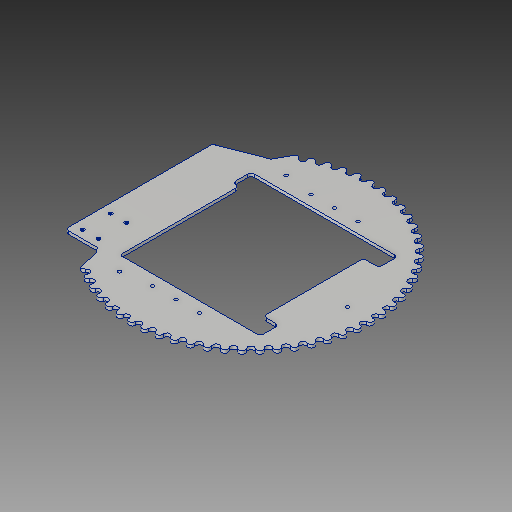
# Autodesk Inventor part: Bearing Plate
Saved by Autodesk Inventor 2019.4 (Build 234330000, 330)
## iProperties
Created: 2020-01-22
Part Number: Bearing Plate
Material: Aluminum 6061
Document SubType Name: Modeling
Designer: admin
Density: 2.7 g/cm^3
Appearance: Aluminum - Flat
Mass: 922.466 g
Surface Area: 1512.08 cm^2
Volume: 341.654 cm^3
Author: admin
Autodesk Inventor part; units mm, degrees
ref_plane "YZ Plane" through (0, 0, 0) normal (1, 0, 0) x (0, 1, 0)
ref_plane "XZ Plane" through (0, 0, 0) normal (0, 1, 0) x (-1, 0, 0)
ref_plane "XY Plane" through (0, 0, 0) normal (0, 0, 1) x (1, 0, 0)
sketch "Sketch1" plane through (0, 0, 0) normal (0, 1, 0) x (-1, 0, 0)
  arc A0 (63.1453, -163.2105) -> (129.2323, 118) centre (0, 0) ccw construction
  circle A1 centre (0, 0) radius 101.6 construction
  line L0 (-100.2, 110.3) -> (100.2, 110.3)
  line L1 (100.2, 110.3) -> (100.2, -110.3)
  line L2 (100.2, -110.3) -> (-100.2, -110.3)
  line L3 (-100.2, -110.3) -> (-100.2, 110.3)
  line L4 (-100.2, 110.3) -> (100.2, -110.3) construction
  line L5 (100.2, 110.3) -> (-100.2, -110.3) construction
  line L6 (180, 118) -> (180, -118)
  line L7 (180, -118) -> (63.1453, -163.2105)
  line L8 (180, 0) -> (0, 0)
  line L9 (180, 118) -> (129.2323, 118)
  arc A2 (129.2323, 118) -> (63.1453, -163.2105) centre (0, 0) ccw
  dimension "d0" = 350
  dimension "d1" = 203.2
  dimension "d4" = 220.6
  dimension "d5" = 200.4
  dimension "d6" = 180
  dimension "d7" = 118
  constraints: 20 end point, 4 point on circle, 3 centre point, 3 midpoint, 2 coincident, 2 horizontal, 2 parallel, 2 perpendicular, 1 tangent, 1 vertical
  measures "d0" diameter of A0
  measures "d1" diameter of A1
  measures "d4" distance of L2.end L0.start
  measures "d5" distance of L0.start L0.end
  measures "d6" distance from line of point (0, 0) L6
  measures "d7" distance from line of point (0, 0) L9
extrude "Extrusion1" add sketch "Sketch1" along normal blind 5
sketch "Sketch2" plane through (0, 0, 0) normal (0, -1, 0) x (1, 0, 0)
  circle A0 centre (-165.208, 60.275) radius 2.0193 construction
  circle A1 centre (-165.208, 105.1064) radius 2.0193 construction
  circle A2 centre (-139.808, 105.1064) radius 2.0193 construction
  circle A3 centre (-139.808, 60.275) radius 2.0193 construction
  circle A4 centre (-165.208, 105.1064) radius 3
  circle A5 centre (-139.808, 105.1064) radius 3
  circle A6 centre (-139.808, 60.275) radius 3
  circle A7 centre (-165.208, 60.275) radius 3
  point P0 (0, 0)
  dimension "d75" = 6
  dimension "d76" = 6
  dimension "d77" = 6
  dimension "d78" = 6
  constraints: 4 centre point, 4 coincident
  measures "d75" diameter of A4
  measures "d76" diameter of A5
  measures "d77" diameter of A6
  measures "d78" diameter of A7
extrude "Extrusion2" cut sketch "Sketch2" against normal through all
chamfer "Chamfer1" distance 3 angle 45 4 edges at (-168.208, 0, 60.275) (-142.808, 0, 60.275) (-142.808, 0, 105.1064) (-168.208, 0, 105.1064)
sketch "Sketch3" plane through (0, 5, 0) normal (0, 1, 0) x (1, 0, 0)
  line L0 (154.73, 0) -> (-77.365, -134.0001) construction
  line L1 (-77.365, -134.0001) -> (-77.365, 134.0001) construction
  line L2 (-77.365, 134.0001) -> (154.73, 0) construction
  circle A0 centre (-77.365, 134.0001) radius 2.75
  circle A1 centre (-77.365, -134.0001) radius 2.75
  circle A2 centre (154.73, 0) radius 2.75
  point P0 (0, 0)
  point P1 (0, 0)
  dimension "d17" = 268.0002
  dimension "d18" = 5.5
  dimension "d19" = 5.5
  dimension "d20" = 5.5
  dimension "d23" = 154.73
  constraints: 6 end point, 4 coincident, 3 centre point, 1 vertical, 7 other
  measures "d17" distance of L1.end L0.start
  measures "d18" diameter of A0
  measures "d19" diameter of A1
  measures "d20" diameter of A2
  measures "d23" distance of A2.centre point (0, 0)
extrude "Extrusion3" cut sketch "Sketch3" against normal through all
sketch "Sketch4" plane through (0, 5, 0) normal (0, 1, 0) x (1, 0, 0)
  circle A0 centre (0, 0) radius 191.0078 construction
  arc A1 (190.8769, -4.9983) -> (190.3537, -14.9812) centre (190.746, -9.9966) ccw
  arc A2 (190.746, -9.9966) -> (201.0078, 0) centre (191.0078, 0) ccw
  arc A3 (199.9066, -21.011) -> (190.746, -9.9966) centre (189.9614, -19.9657) ccw
  line L0 (0, 0) -> (199.9066, -21.011) construction
  arc A4 (189.3088, -24.923) -> (193.6558, -29.9343) centre (188.6561, -29.8802) ccw construction
  line L1 (0, 0) -> (201.0078, 0)
  arc A5 (195.7441, 9.8581) -> (190.8769, 4.9983) centre (190.746, 9.9966) ccw construction
  arc A6 (189.3088, -24.923) -> (190.3537, -14.9812) centre (189.9614, -19.9657) ccw
  arc A7 (190.8769, -4.9983) -> (190.8769, 4.9983) centre (191.0078, 0) ccw
  arc A8 (-129.2323, -118) -> (-63.1453, 163.2105) centre (0, 0) ccw projected
  line L2 (196.0078, 0) -> (175, 0)
  line L3 (194.934, -20.4884) -> (174.0413, -18.2925)
  arc A9 (201.0078, 0) -> (190.746, 9.9966) centre (191.0078, 0) ccw
  arc A10 (190.746, 9.9966) -> (199.9066, 21.011) centre (189.9614, 19.9657) ccw
  arc A11 (199.9066, 21.011) -> (188.6561, 29.8802) centre (189.9614, 19.9657) ccw
  arc A12 (188.6561, 29.8802) -> (196.6152, 41.7919) centre (186.8338, 39.7127) ccw
  arc A13 (196.6152, 41.7919) -> (184.4993, 49.4364) centre (186.8338, 39.7127) ccw
  arc A14 (184.4993, 49.4364) -> (191.1697, 62.1148) centre (181.6592, 59.0246) ccw
  arc A15 (191.1697, 62.1148) -> (178.3211, 68.4511) centre (181.6592, 59.0246) ccw
  arc A16 (178.3211, 68.4511) -> (183.6297, 81.7572) centre (174.4943, 77.6899) ccw
  arc A17 (183.6297, 81.7572) -> (170.1892, 86.7157) centre (174.4943, 77.6899) ccw
  arc A18 (170.1892, 86.7157) -> (174.0778, 100.5039) centre (165.4176, 95.5039) ccw
  arc A19 (174.0778, 100.5039) -> (160.1926, 104.0303) centre (165.4176, 95.5039) ccw
  arc A20 (160.1926, 104.0303) -> (162.6187, 118.1494) centre (154.5285, 112.2715) ccw
  arc A21 (162.6187, 118.1494) -> (148.4409, 120.2051) centre (154.5285, 112.2715) ccw
  arc A22 (148.4409, 120.2051) -> (149.3779, 134.5004) centre (141.9464, 127.8091) ccw
  arc A23 (149.3779, 134.5004) -> (135.0629, 135.0629) centre (141.9464, 127.8091) ccw
  arc A24 (135.0629, 135.0629) -> (134.5004, 149.3779) centre (127.8091, 141.9464) ccw
  arc A25 (134.5004, 149.3779) -> (120.2051, 148.4409) centre (127.8091, 141.9464) ccw
  arc A26 (120.2051, 148.4409) -> (118.1494, 162.6187) centre (112.2715, 154.5285) ccw
  arc A27 (118.1494, 162.6187) -> (104.0303, 160.1926) centre (112.2715, 154.5285) ccw
  arc A28 (104.0303, 160.1926) -> (100.5039, 174.0778) centre (95.5039, 165.4176) ccw
  arc A29 (100.5039, 174.0778) -> (86.7157, 170.1892) centre (95.5039, 165.4176) ccw
  arc A30 (86.7157, 170.1892) -> (81.7572, 183.6297) centre (77.6899, 174.4943) ccw
  arc A31 (81.7572, 183.6297) -> (68.4511, 178.3211) centre (77.6899, 174.4943) ccw
  arc A32 (68.4511, 178.3211) -> (62.1148, 191.1697) centre (59.0246, 181.6592) ccw
  arc A33 (62.1148, 191.1697) -> (49.4364, 184.4993) centre (59.0246, 181.6592) ccw
  arc A34 (49.4364, 184.4993) -> (41.7919, 196.6152) centre (39.7127, 186.8338) ccw
  arc A35 (41.7919, 196.6152) -> (29.8802, 188.6561) centre (39.7127, 186.8338) ccw
  arc A36 (29.8802, 188.6561) -> (21.011, 199.9066) centre (19.9657, 189.9614) ccw
  arc A37 (21.011, 199.9066) -> (9.9966, 190.746) centre (19.9657, 189.9614) ccw
  arc A38 (9.9966, 190.746) -> (0, 201.0078) centre (0, 191.0078) ccw
  arc A39 (0, 201.0078) -> (-9.9966, 190.746) centre (0, 191.0078) ccw
  arc A40 (-9.9966, 190.746) -> (-21.011, 199.9066) centre (-19.9657, 189.9614) ccw
  arc A41 (-21.011, 199.9066) -> (-29.8802, 188.6561) centre (-19.9657, 189.9614) ccw
  arc A42 (-29.8802, 188.6561) -> (-41.7919, 196.6152) centre (-39.7127, 186.8338) ccw
  arc A43 (-41.7919, 196.6152) -> (-49.4364, 184.4993) centre (-39.7127, 186.8338) ccw
  arc A44 (-49.4364, 184.4993) -> (-62.1148, 191.1697) centre (-59.0246, 181.6592) ccw
  arc A45 (-62.1148, 191.1697) -> (-68.4511, 178.3211) centre (-59.0246, 181.6592) ccw
  arc A46 (-68.4511, 178.3211) -> (-81.7572, 183.6297) centre (-77.6899, 174.4943) ccw
  arc A47 (-81.7572, 183.6297) -> (-86.7157, 170.1892) centre (-77.6899, 174.4943) ccw
  arc A48 (-86.7157, 170.1892) -> (-100.5039, 174.0778) centre (-95.5039, 165.4176) ccw
  arc A49 (196.3819, -42.8749) -> (188.4886, -30.9195) centre (186.6121, -40.7419) ccw
  arc A50 (188.4886, -30.9195) -> (199.7878, -22.1125) centre (189.8485, -21.0124) ccw
  arc A51 (190.4734, -64.2183) -> (183.9432, -51.4672) centre (180.9975, -61.0235) ccw
  arc A52 (183.9432, -51.4672) -> (196.1426, -43.9566) centre (186.3847, -41.7698) ccw
  arc A53 (182.2528, -84.7822) -> (177.165, -71.39) centre (173.1859, -80.5643) ccw
  arc A54 (177.165, -71.39) -> (190.1166, -65.2671) centre (180.6584, -62.0201) ccw
  arc A55 (171.82, -104.3169) -> (168.2362, -90.4464) centre (163.272, -99.1272) ccw
  arc A56 (168.2362, -90.4464) -> (181.7828, -85.7854) centre (172.7392, -81.5176) ccw
  arc A57 (159.3014, -122.5854) -> (157.2653, -108.4048) centre (151.3763, -116.4868) ccw
  arc A58 (157.2653, -108.4048) -> (171.2424, -105.2623) centre (162.7232, -100.0256) ccw
  arc A59 (144.8492, -139.3658) -> (144.3854, -125.0473) centre (137.643, -132.4325) ccw
  arc A60 (144.3854, -125.0473) -> (158.6234, -123.4615) centre (150.732, -117.3194) ccw
  arc A61 (128.6386, -154.4546) -> (129.7528, -140.1719) centre (122.239, -146.7706) ccw
  arc A62 (129.7528, -140.1719) -> (144.0788, -140.1621) centre (136.911, -133.1891) ccw
  arc A63 (110.8666, -167.6685) -> (113.5452, -153.5951) centre (105.3511, -159.3271) ccw
  arc A64 (113.5452, -153.5951) -> (127.7854, -155.1612) centre (121.4282, -147.4421) ccw
  arc A65 (91.7488, -178.8471) -> (95.9594, -165.1537) centre (87.1844, -169.9495) ccw
  arc A66 (95.9594, -165.1537) -> (109.9408, -168.277) centre (104.4713, -159.9053) ccw
  arc A67 (71.5173, -187.8547) -> (77.2087, -174.7077) centre (67.9594, -178.5091) ccw
  arc A68 (77.2087, -174.7077) -> (90.7617, -179.35) centre (86.2464, -170.4275) ccw
  arc A69 (50.4177, -194.582) -> (57.5208, -182.1409) centre (47.9095, -184.9017) ccw
  arc A70 (57.5208, -182.1409) -> (70.4809, -188.246) centre (66.9745, -178.8809) ccw
  arc A71 (28.7061, -198.9474) -> (37.1347, -187.3632) centre (27.278, -189.0499) ccw
  arc A72 (37.1347, -187.3632) -> (49.3445, -194.857) centre (46.8896, -185.163) ccw
  arc A73 (6.646, -200.8979) -> (16.2978, -190.3112) centre (6.3154, -190.9033) ccw
  arc A74 (16.2978, -190.3112) -> (27.6091, -199.1026) centre (26.2356, -189.1974) ccw
  arc A75 (-15.4948, -200.4097) -> (-4.7369, -190.949) centre (-14.7239, -190.4394) ccw
  arc A76 (-4.7369, -190.949) -> (5.5386, -200.9314) centre (5.2631, -190.9352) ccw
  arc A77 (-37.4474, -197.4887) -> (-25.7141, -189.269) centre (-35.5844, -187.6638) ccw
  arc A78 (-25.7141, -189.269) -> (-16.5991, -200.3212) centre (-15.7733, -190.3554) ccw
  arc A79 (-58.9455, -192.1706) -> (-46.3792, -185.2915) centre (-56.013, -182.6102) ccw
  arc A80 (-46.3792, -185.2915) -> (-38.5353, -197.2794) centre (-36.6182, -187.4648) ccw
  arc A81 (-79.7281, -184.5198) -> (-66.4813, -179.0648) centre (-75.7617, -175.34) ccw
  arc A82 (-66.4813, -179.0648) -> (-60.0038, -191.8428) centre (-57.0186, -182.2988) ccw
  arc A83 (-99.5429, -174.6291) -> (-85.7764, -170.6645) centre (-94.5907, -165.9414) ccw
  arc A84 (-85.7764, -170.6645) -> (-80.7439, -184.0775) centre (-76.7269, -174.9198) ccw
  arc A85 (-118.1494, -162.6187) -> (-104.0303, -160.1926) centre (-112.2715, -154.5285) ccw
  arc A86 (-104.0303, -160.1926) -> (-100.5039, -174.0778) centre (-95.5039, -165.4176) ccw
  dimension "d24" = 5
  dimension "d28" = 5
  dimension "d30" = 6
  dimension "d31" = 5
  dimension "d32" = 5
  dimension "d33" = 5
  dimension "d45" = 120
  dimension "d49" = 120
  constraints: 179 point on circle, 86 centre point, 8 end point, 4 equal radius, 4 point on line, 3 coincident, 1 horizontal, 275 other
  measures "d24" radius of A1
  measures "d28" radius of A4
  measures "d30" angle of L0 L1
  measures "d31" radius of A5
  measures "d32" radius of A6
  measures "d33" radius of A7
extrude "Extrusion4" add sketch "Sketch4" against normal up to surface (5 mm away)
pattern_circular "Circular Pattern1" count 41 over 240 about axis through (0, -10, 0) along (0, 1, 0) of "Extrusion4" both ways yes
sketch "Sketch5" plane through (0, 5, 0) normal (0, 1, 0) x (1, 0, 0)
  line L0 (-115.2105, -158.5736) -> (-122.0328, -125.4312)
  arc A0 (-91.1098, 167.8034) -> (-98.0039, 169.7477) centre (-95.5039, 165.4176) ccw projected
  line L1 (-98.0039, 169.7477) -> (-112.1506, 144.2506)
  line L2 (-88.554, 153.38) -> (-180, 118) projected
  line L3 (-88.554, 153.38) -> (-98.0039, 169.7477)
  arc A1 (-129.2323, -118) -> (-102.8624, -141.578) centre (0, 0) ccw projected
  line L4 (-115.2105, -158.5736) -> (-102.8624, -141.578) projected
  dimension "d51" = 25
  dimension "d52" = 25
  constraints: 6 end point, 1 point on circle, 1 point on line
  measures "d51" distance from line of L4 L0.end
  measures "d52" distance from line of L3 L1.end
extrude "Extrusion5" add sketch "Sketch5" against normal up to surface (5 mm away)
sketch "Sketch6" plane through (0, 5, 0) normal (0, 1, 0) x (1, 0, 0)
  line L0 (-100.2, -110.3) -> (-100.2, 110.3) projected
  line L1 (-100.2, 110.3) -> (-110.2, 110.3)
  line L2 (-110.2, 110.3) -> (-110.2, 80.3)
  line L3 (-110.2, 80.3) -> (-100.2, 80.3)
  point P0 (0, 0)
  dimension "d59" = 30
  dimension "d60" = 10
  constraints: 6 end point, 2 perpendicular, 1 horizontal, 1 point on line
  measures "d59" distance of L1.end L2.end
  measures "d60" distance of L2.end L3.end
extrude "Extrusion6" cut sketch "Sketch6" against normal through all
sketch "Sketch10" plane through (0, 5, 0) normal (0, 1, 0) x (1, 0, 0)
  line L0 (100.2, -110.3) -> (125.2, -110.3)
  line L1 (125.2, -110.3) -> (125.2, -80.3)
  line L2 (125.2, -80.3) -> (100.2, -80.3)
  line L3 (100.2, -110.3) -> (100.2, 110.3) projected
  point P0 (0, 0)
  dimension "d81" = 30
  dimension "d82" = 25
  constraints: 6 end point, 2 perpendicular, 1 horizontal, 1 point on line
  measures "d81" distance of L0.end L1.end
  measures "d82" distance of L0.start L0.end
extrude "Extrusion8" cut sketch "Sketch10" against normal through all
mirror "Mirror1" about plane through (0, 0, 0) normal (0, 0, 1) of "Extrusion8"
fillet "Fillet1" radius 5 9 edges at (-110.2, 2.5, -110.3) (-110.2, 2.5, -80.3) (-100.2, 2.5, -80.3) (100.2, 2.5, 80.3) (125.2, 2.5, 80.3) (125.2, 2.5, 110.3) (100.2, 2.5, -80.3) (125.2, 2.5, -80.3) (125.2, 2.5, -110.3)
fillet "Fillet2" radius 2 2 edges at (-115.2105, 2.5, 158.5736) (-98.0039, 2.5, -169.7477)
fillet "Fillet3" radius 2.5 1 edges at (-100.2, 2.5, 110.3)
fillet "Fillet4" radius 5 2 edges at (-180, 2.5, 118) (-180, 2.5, -118)
sketch "Sketch8" plane through (0, 5, 0) normal (0, 1, 0) x (1, 0, 0)
  arc A0 (-100.2, 75.3) -> (-105.2, 80.3) centre (-105.2, 75.3) ccw projected
  arc A1 (-110.2, 85.3) -> (-105.2, 80.3) centre (-105.2, 85.3) ccw projected
  line L0 (-110.2, 85.3) -> (-110.2, 105.3) projected
  arc A2 (-105.2, 110.3) -> (-110.2, 105.3) centre (-105.2, 105.3) ccw projected
  line L1 (-105.2, 110.3) -> (120.2, 110.3) projected
  line L2 (100.2, 75.3) -> (100.2, -75.3) projected
  line L3 (120.2, -110.3) -> (-97.7, -110.3) projected
  arc A3 (-100.2, -107.8) -> (-97.7, -110.3) centre (-97.7, -107.8) ccw projected
  line L4 (-100.2, -107.8) -> (-100.2, 75.3) projected
  circle A4 centre (154.73, 0) radius 2.75 projected
  circle A5 centre (-77.365, 134.0001) radius 2.75 projected
  circle A6 centre (-77.365, -134.0001) radius 2.75 projected
  arc A7 (-176.8042, 119.2365) -> (-180, 114.5733) centre (-175, 114.5733) ccw projected
  line L5 (-180, 114.5733) -> (-180, -113) projected
  arc A8 (-180, -113) -> (-175, -118) centre (-175, -113) ccw projected
  line L6 (-175, -118) -> (-129.2323, -118) projected
  arc A9 (-129.2323, -118) -> (-122.0328, -125.4312) centre (0, 0) ccw projected
  line L7 (-115.3906, -157.6983) -> (-122.0328, -125.4312) projected
  arc A10 (-115.3906, -157.6983) -> (-114.2052, -159.1395) centre (-113.4317, -157.2951) ccw projected
  arc A11 (-114.2052, -159.1395) -> (-108.1509, -157.3605) centre (-112.2715, -154.5285) ccw projected
  arc A12 (-99.7671, -162.8051) -> (-108.1509, -157.3605) centre (-104.0303, -160.1926) ccw projected
  arc A13 (-99.7671, -162.8051) -> (-91.1098, -167.8034) centre (-95.5039, -165.4176) ccw projected
  arc A14 (-82.2028, -172.3417) -> (-91.1098, -167.8034) centre (-86.7157, -170.1892) ccw projected
  arc A15 (-82.2028, -172.3417) -> (-73.0705, -176.4077) centre (-77.6899, -174.4943) ccw projected
  arc A16 (-63.7378, -179.9901) -> (-73.0705, -176.4077) centre (-68.4511, -178.3211) ccw projected
  arc A17 (-63.7378, -179.9901) -> (-54.2305, -183.0792) centre (-59.0246, -181.6592) ccw projected
  arc A18 (-44.5746, -185.6665) -> (-54.2305, -183.0792) centre (-49.4364, -184.4993) ccw projected
  arc A19 (-44.5746, -185.6665) -> (-34.7965, -187.745) centre (-39.7127, -186.8338) ccw projected
  arc A20 (-24.923, -189.3088) -> (-34.7965, -187.745) centre (-29.8802, -188.6561) ccw projected
  arc A21 (-24.923, -189.3088) -> (-14.9812, -190.3537) centre (-19.9657, -189.9614) ccw projected
  arc A22 (-4.9983, -190.8769) -> (-14.9812, -190.3537) centre (-9.9966, -190.746) ccw projected
  arc A23 (-4.9983, -190.8769) -> (4.9983, -190.8769) centre (0, -191.0078) ccw projected
  arc A24 (14.9812, -190.3537) -> (4.9983, -190.8769) centre (9.9966, -190.746) ccw projected
  arc A25 (14.9812, -190.3537) -> (24.923, -189.3088) centre (19.9657, -189.9614) ccw projected
  arc A26 (34.7965, -187.745) -> (24.923, -189.3088) centre (29.8802, -188.6561) ccw projected
  arc A27 (34.7965, -187.745) -> (44.5746, -185.6665) centre (39.7127, -186.8338) ccw projected
  arc A28 (54.2305, -183.0792) -> (44.5746, -185.6665) centre (49.4364, -184.4993) ccw projected
  arc A29 (54.2305, -183.0792) -> (63.7378, -179.9901) centre (59.0246, -181.6592) ccw projected
  arc A30 (73.0705, -176.4077) -> (63.7378, -179.9901) centre (68.4511, -178.3211) ccw projected
  arc A31 (73.0705, -176.4077) -> (82.2028, -172.3417) centre (77.6899, -174.4943) ccw projected
  arc A32 (91.1098, -167.8034) -> (82.2028, -172.3417) centre (86.7157, -170.1892) ccw projected
  arc A33 (91.1098, -167.8034) -> (99.7671, -162.8051) centre (95.5039, -165.4176) ccw projected
  arc A34 (108.1509, -157.3605) -> (99.7671, -162.8051) centre (104.0303, -160.1926) ccw projected
  arc A35 (108.1509, -157.3605) -> (116.2383, -151.4847) centre (112.2715, -154.5285) ccw projected
  arc A36 (124.0071, -145.1937) -> (116.2383, -151.4847) centre (120.2051, -148.4409) ccw projected
  arc A37 (124.0071, -145.1937) -> (131.436, -138.5046) centre (127.8091, -141.9464) ccw projected
  arc A38 (138.5046, -131.436) -> (131.436, -138.5046) centre (135.0629, -135.0629) ccw projected
  arc A39 (138.5046, -131.436) -> (145.1937, -124.0071) centre (141.9464, -127.8091) ccw projected
  arc A40 (151.4847, -116.2383) -> (145.1937, -124.0071) centre (148.4409, -120.2051) ccw projected
  arc A41 (151.4847, -116.2383) -> (157.3605, -108.1509) centre (154.5285, -112.2715) ccw projected
  arc A42 (162.8051, -99.7671) -> (157.3605, -108.1509) centre (160.1926, -104.0303) ccw projected
  arc A43 (162.8051, -99.7671) -> (167.8034, -91.1098) centre (165.4176, -95.5039) ccw projected
  arc A44 (172.3417, -82.2028) -> (167.8034, -91.1098) centre (170.1892, -86.7157) ccw projected
  arc A45 (172.3417, -82.2028) -> (176.4077, -73.0705) centre (174.4943, -77.6899) ccw projected
  arc A46 (179.9901, -63.7378) -> (176.4077, -73.0705) centre (178.3211, -68.4511) ccw projected
  arc A47 (179.9901, -63.7378) -> (183.0792, -54.2305) centre (181.6592, -59.0246) ccw projected
  arc A48 (185.6665, -44.5746) -> (183.0792, -54.2305) centre (184.4993, -49.4364) ccw projected
  arc A49 (185.6665, -44.5746) -> (187.745, -34.7965) centre (186.8338, -39.7127) ccw projected
  arc A50 (189.3088, -24.923) -> (187.745, -34.7965) centre (188.6561, -29.8802) ccw projected
  arc A51 (189.3088, -24.923) -> (190.3537, -14.9812) centre (189.9614, -19.9657) ccw projected
  arc A52 (190.8769, -4.9983) -> (190.3537, -14.9812) centre (190.746, -9.9966) ccw projected
  arc A53 (190.8769, -4.9983) -> (190.8769, 4.9983) centre (191.0078, 0) ccw projected
  arc A54 (190.3537, 14.9812) -> (190.8769, 4.9983) centre (190.746, 9.9966) ccw projected
  arc A55 (190.3537, 14.9812) -> (189.3088, 24.923) centre (189.9614, 19.9657) ccw projected
  arc A56 (187.745, 34.7965) -> (189.3088, 24.923) centre (188.6561, 29.8802) ccw projected
  arc A57 (187.745, 34.7965) -> (185.6665, 44.5746) centre (186.8338, 39.7127) ccw projected
  arc A58 (183.0792, 54.2305) -> (185.6665, 44.5746) centre (184.4993, 49.4364) ccw projected
  arc A59 (183.0792, 54.2305) -> (179.9901, 63.7378) centre (181.6592, 59.0246) ccw projected
  arc A60 (176.4077, 73.0705) -> (179.9901, 63.7378) centre (178.3211, 68.4511) ccw projected
  arc A61 (176.4077, 73.0705) -> (172.3417, 82.2028) centre (174.4943, 77.6899) ccw projected
  arc A62 (167.8034, 91.1098) -> (172.3417, 82.2028) centre (170.1892, 86.7157) ccw projected
  arc A63 (167.8034, 91.1098) -> (162.8051, 99.7671) centre (165.4176, 95.5039) ccw projected
  arc A64 (157.3605, 108.1509) -> (162.8051, 99.7671) centre (160.1926, 104.0303) ccw projected
  arc A65 (157.3605, 108.1509) -> (151.4847, 116.2383) centre (154.5285, 112.2715) ccw projected
  arc A66 (145.1937, 124.0071) -> (151.4847, 116.2383) centre (148.4409, 120.2051) ccw projected
  arc A67 (145.1937, 124.0071) -> (138.5046, 131.436) centre (141.9464, 127.8091) ccw projected
  arc A68 (131.436, 138.5046) -> (138.5046, 131.436) centre (135.0629, 135.0629) ccw projected
  arc A69 (131.436, 138.5046) -> (124.0071, 145.1937) centre (127.8091, 141.9464) ccw projected
  arc A70 (116.2383, 151.4847) -> (124.0071, 145.1937) centre (120.2051, 148.4409) ccw projected
  arc A71 (116.2383, 151.4847) -> (108.1509, 157.3605) centre (112.2715, 154.5285) ccw projected
  arc A72 (99.7671, 162.8051) -> (108.1509, 157.3605) centre (104.0303, 160.1926) ccw projected
  arc A73 (99.7671, 162.8051) -> (91.1098, 167.8034) centre (95.5039, 165.4176) ccw projected
  arc A74 (82.2028, 172.3417) -> (91.1098, 167.8034) centre (86.7157, 170.1892) ccw projected
  arc A75 (82.2028, 172.3417) -> (73.0705, 176.4077) centre (77.6899, 174.4943) ccw projected
  arc A76 (63.7378, 179.9901) -> (73.0705, 176.4077) centre (68.4511, 178.3211) ccw projected
  arc A77 (63.7378, 179.9901) -> (54.2305, 183.0792) centre (59.0246, 181.6592) ccw projected
  arc A78 (44.5746, 185.6665) -> (54.2305, 183.0792) centre (49.4364, 184.4993) ccw projected
  arc A79 (44.5746, 185.6665) -> (34.7965, 187.745) centre (39.7127, 186.8338) ccw projected
  arc A80 (24.923, 189.3088) -> (34.7965, 187.745) centre (29.8802, 188.6561) ccw projected
  arc A81 (24.923, 189.3088) -> (14.9812, 190.3537) centre (19.9657, 189.9614) ccw projected
  arc A82 (4.9983, 190.8769) -> (14.9812, 190.3537) centre (9.9966, 190.746) ccw projected
  arc A83 (4.9983, 190.8769) -> (-4.9983, 190.8769) centre (0, 191.0078) ccw projected
  arc A84 (-14.9812, 190.3537) -> (-4.9983, 190.8769) centre (-9.9966, 190.746) ccw projected
  arc A85 (-14.9812, 190.3537) -> (-24.923, 189.3088) centre (-19.9657, 189.9614) ccw projected
  arc A86 (-34.7965, 187.745) -> (-24.923, 189.3088) centre (-29.8802, 188.6561) ccw projected
  arc A87 (-34.7965, 187.745) -> (-44.5746, 185.6665) centre (-39.7127, 186.8338) ccw projected
  arc A88 (-54.2305, 183.0792) -> (-44.5746, 185.6665) centre (-49.4364, 184.4993) ccw projected
  arc A89 (-54.2305, 183.0792) -> (-63.7378, 179.9901) centre (-59.0246, 181.6592) ccw projected
  arc A90 (-73.0705, 176.4077) -> (-63.7378, 179.9901) centre (-68.4511, 178.3211) ccw projected
  arc A91 (-73.0705, 176.4077) -> (-82.2028, 172.3417) centre (-77.6899, 174.4943) ccw projected
  arc A92 (-91.1098, 167.8034) -> (-82.2028, 172.3417) centre (-86.7157, 170.1892) ccw projected
  arc A93 (-91.1098, 167.8034) -> (-97.2666, 170.0965) centre (-95.5039, 165.4176) ccw projected
  arc A94 (-97.2666, 170.0965) -> (-98.3104, 169.1953) centre (-96.5615, 168.2249) ccw projected
  line L8 (-98.3104, 169.1953) -> (-112.1506, 144.2506) projected
  line L9 (-112.1506, 144.2506) -> (-176.8042, 119.2365) projected
  line L10 (-185, -113) -> (-185, 114.5733)
  arc A95 (-178.6083, 123.8996) -> (-185, 114.5733) centre (-175, 114.5733) ccw
  line L11 (-178.6083, 123.8996) -> (-115.644, 148.2602)
  line L12 (-115.644, 148.2602) -> (-102.6825, 171.6211)
  arc A96 (-99.0294, 174.7755) -> (-102.6825, 171.6211) centre (-96.5615, 168.2249) ccw
  arc A97 (-86.7157, 170.1892) -> (-99.0294, 174.7755) centre (-95.5039, 165.4176) ccw
  arc A98 (-68.4511, 178.3211) -> (-86.7157, 170.1892) centre (-77.6899, 174.4943) ccw
  arc A99 (-49.4364, 184.4993) -> (-68.4511, 178.3211) centre (-59.0246, 181.6592) ccw
  arc A100 (-29.8802, 188.6561) -> (-49.4364, 184.4993) centre (-39.7127, 186.8338) ccw
  arc A101 (-9.9966, 190.746) -> (-29.8802, 188.6561) centre (-19.9657, 189.9614) ccw
  arc A102 (9.9966, 190.746) -> (-9.9966, 190.746) centre (0, 191.0078) ccw
  arc A103 (29.8802, 188.6561) -> (9.9966, 190.746) centre (19.9657, 189.9614) ccw
  arc A104 (49.4364, 184.4993) -> (29.8802, 188.6561) centre (39.7127, 186.8338) ccw
  arc A105 (68.4511, 178.3211) -> (49.4364, 184.4993) centre (59.0246, 181.6592) ccw
  arc A106 (86.7157, 170.1892) -> (68.4511, 178.3211) centre (77.6899, 174.4943) ccw
  arc A107 (104.0303, 160.1926) -> (86.7157, 170.1892) centre (95.5039, 165.4176) ccw
  arc A108 (120.2051, 148.4409) -> (104.0303, 160.1926) centre (112.2715, 154.5285) ccw
  arc A109 (135.0629, 135.0629) -> (120.2051, 148.4409) centre (127.8091, 141.9464) ccw
  arc A110 (148.4409, 120.2051) -> (135.0629, 135.0629) centre (141.9464, 127.8091) ccw
  arc A111 (160.1926, 104.0303) -> (148.4409, 120.2051) centre (154.5285, 112.2715) ccw
  arc A112 (170.1892, 86.7157) -> (160.1926, 104.0303) centre (165.4176, 95.5039) ccw
  arc A113 (178.3211, 68.4511) -> (170.1892, 86.7157) centre (174.4943, 77.6899) ccw
  arc A114 (184.4993, 49.4364) -> (178.3211, 68.4511) centre (181.6592, 59.0246) ccw
  arc A115 (188.6561, 29.8802) -> (184.4993, 49.4364) centre (186.8338, 39.7127) ccw
  arc A116 (190.746, 9.9966) -> (188.6561, 29.8802) centre (189.9614, 19.9657) ccw
  arc A117 (190.746, -9.9966) -> (190.746, 9.9966) centre (191.0078, 0) ccw
  arc A118 (188.6561, -29.8802) -> (190.746, -9.9966) centre (189.9614, -19.9657) ccw
  arc A119 (184.4993, -49.4364) -> (188.6561, -29.8802) centre (186.8338, -39.7127) ccw
  arc A120 (178.3211, -68.4511) -> (184.4993, -49.4364) centre (181.6592, -59.0246) ccw
  arc A121 (170.1892, -86.7157) -> (178.3211, -68.4511) centre (174.4943, -77.6899) ccw
  arc A122 (160.1926, -104.0303) -> (170.1892, -86.7157) centre (165.4176, -95.5039) ccw
  arc A123 (148.4409, -120.2051) -> (160.1926, -104.0303) centre (154.5285, -112.2715) ccw
  arc A124 (135.0629, -135.0629) -> (148.4409, -120.2051) centre (141.9464, -127.8091) ccw
  arc A125 (120.2051, -148.4409) -> (135.0629, -135.0629) centre (127.8091, -141.9464) ccw
  arc A126 (104.0303, -160.1926) -> (120.2051, -148.4409) centre (112.2715, -154.5285) ccw
  arc A127 (86.7157, -170.1892) -> (104.0303, -160.1926) centre (95.5039, -165.4176) ccw
  arc A128 (68.4511, -178.3211) -> (86.7157, -170.1892) centre (77.6899, -174.4943) ccw
  arc A129 (49.4364, -184.4993) -> (68.4511, -178.3211) centre (59.0246, -181.6592) ccw
  arc A130 (29.8802, -188.6561) -> (49.4364, -184.4993) centre (39.7127, -186.8338) ccw
  arc A131 (9.9966, -190.746) -> (29.8802, -188.6561) centre (19.9657, -189.9614) ccw
  arc A132 (-9.9966, -190.746) -> (9.9966, -190.746) centre (0, -191.0078) ccw
  arc A133 (-29.8802, -188.6561) -> (-9.9966, -190.746) centre (-19.9657, -189.9614) ccw
  arc A134 (-49.4364, -184.4993) -> (-29.8802, -188.6561) centre (-39.7127, -186.8338) ccw
  arc A135 (-68.4511, -178.3211) -> (-49.4364, -184.4993) centre (-59.0246, -181.6592) ccw
  arc A136 (-86.7157, -170.1892) -> (-68.4511, -178.3211) centre (-77.6899, -174.4943) ccw
  arc A137 (-104.0303, -160.1926) -> (-86.7157, -170.1892) centre (-95.5039, -165.4176) ccw
  arc A138 (-116.1388, -163.7505) -> (-104.0303, -160.1926) centre (-112.2715, -154.5285) ccw
  arc A139 (-120.288, -158.7065) -> (-116.1388, -163.7505) centre (-113.4317, -157.2951) ccw
  line L13 (-120.288, -158.7065) -> (-126.6228, -127.9323)
  arc A140 (-131.4192, -123) -> (-126.6228, -127.9323) centre (0, 0) ccw
  line L14 (-131.4192, -123) -> (-175, -123)
  arc A141 (-185, -113) -> (-175, -123) centre (-175, -113) ccw
  arc A142 (-95.2, 75.3) -> (-105.2, 85.3) centre (-105.2, 75.3) ccw
  line L15 (-105.2, 85.3) -> (-105.2, 105.3)
  line L16 (-105.2, 105.3) -> (95.2, 105.3)
  line L17 (95.2, 105.3) -> (95.2, -105.3)
  line L18 (95.2, -105.3) -> (-95.2, -105.3)
  line L19 (-95.2, -105.3) -> (-95.2, 75.3)
  arc A143 (100.2, -75.3) -> (105.2, -80.3) centre (105.2, -75.3) ccw projected
  line L20 (105.2, -80.3) -> (120.2, -80.3) projected
  arc A144 (125.2, -85.3) -> (120.2, -80.3) centre (120.2, -85.3) ccw projected
  line L21 (125.2, -85.3) -> (125.2, -105.3) projected
  arc A145 (120.2, -110.3) -> (125.2, -105.3) centre (120.2, -105.3) ccw projected
  line L22 (125.2, 105.3) -> (125.2, 85.3) projected
  line L23 (120.2, 80.3) -> (105.2, 80.3) projected
  arc A146 (105.2, 80.3) -> (100.2, 75.3) centre (105.2, 75.3) ccw projected
  arc A147 (125.2, 105.3) -> (120.2, 110.3) centre (120.2, 105.3) ccw projected
  arc A148 (120.2, 80.3) -> (125.2, 85.3) centre (120.2, 85.3) ccw projected
  dimension "d69" = 5
  dimension "d70" = 5
  constraints: 96 point on circle, 48 centre point, 20 end point, 56 other
  measures "d69" distance between parallel lines of L5 L10
  measures "d70" distance between parallel lines of L4 L19
sketch "Sketch9" plane through (0, 5, 0) normal (0, 1, 0) x (1, 0, 0)
  circle A0 centre (-30.7, -127.3) radius 2.75 projected
  circle A1 centre (6.8, -127.3) radius 2.75 projected
  circle A2 centre (44.3, -127.3) radius 2.75 projected
  circle A3 centre (-30.7, 127.3) radius 2.75 projected
  circle A4 centre (6.8, 127.3) radius 2.75 projected
  circle A5 centre (44.3, 127.3) radius 2.75 projected
  point P0 (0, 0)
extrude "Extrusion7" cut sketch "Sketch9" against normal through all
body "Solid1"
